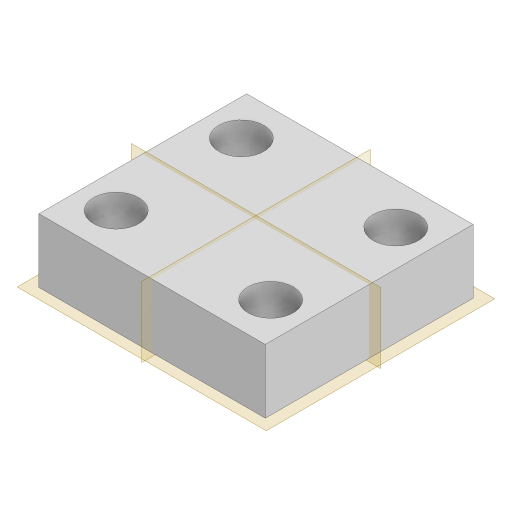
# Autodesk Inventor part: Крепление мотора2
Saved by Autodesk Inventor 2023.2 (Build 272271030, 271C)
## iProperties
Created: 2024-12-17
Part Number: Крепление мотора2
Material: Типовые
Document SubType Name: Modeling
Designer: I9232
Density: 1 g/cm^3
Appearance: По умолчанию
Author: I9232
Autodesk Inventor part; units mm, degrees
sketch "Эскиз1" plane through (0, 0, 0) normal (0, 1, 0) x (-1, 0, 0)
  line L0 (21.25, 19.5) -> (-21.25, 19.5)
  line L1 (-21.25, 19.5) -> (-21.25, -19.5)
  line L2 (-21.25, -19.5) -> (21.25, -19.5)
  line L3 (21.25, -19.5) -> (21.25, 19.5)
  line L4 (21.25, 19.5) -> (-21.25, -19.5) construction
  line L5 (-21.25, 19.5) -> (21.25, -19.5) construction
  circle A0 centre (-14.5, -11.75) radius 4.25
  line L6 (0, -19.5) -> (0, 19.5) construction
  line L7 (-21.25, 0) -> (21.25, 0) construction
  circle A1 centre (14.5, -11.75) radius 4.25
  circle A2 centre (-14.5, 11.75) radius 4.25
  circle A3 centre (14.5, 11.75) radius 4.25
  point P0 (0, 0)
  dimension "d0" = 39
  dimension "d1" = 42.5
  dimension "d2" = 8.5
  dimension "d3" = 6.75
  dimension "d4" = 7.75
  constraints: 16 end point, 6 midpoint, 4 centre point, 3 symmetric about line, 2 parallel, 1 horizontal, 1 perpendicular, 3 other
  measures "d0" distance of L0.end L1.end
  measures "d1" distance of L1.end L2.end
  measures "d2" diameter of A0
  measures "d3" distance from line of L1 A0.centre
  measures "d4" distance from line of L2 A0.centre
extrude "Выдавливание1" add sketch "Эскиз1" along normal blind 12
